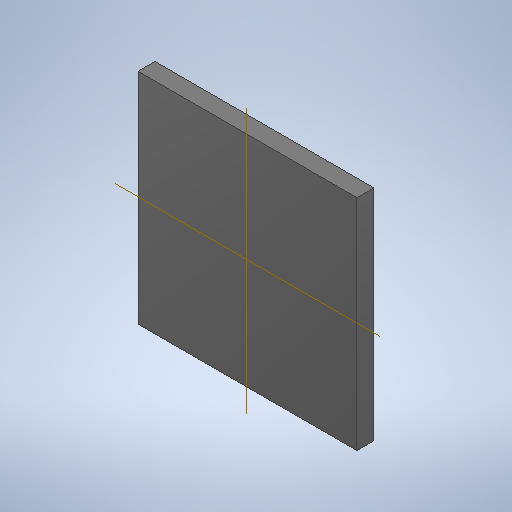
# Autodesk Inventor part: display
Saved by Autodesk Inventor 2025.1 (Build 291241000, 241)
## iProperties
Created: 2024-10-28
Part Number: display
Material: 일반
Document SubType Name: Modeling
Designer: gmsee
Density: 1 g/cm^3
Appearance: 기본값
Author: gmsee
Autodesk Inventor part; units mm, degrees
ref_plane "YZ Plane" through (0, 0, 0) normal (1, 0, 0) x (0, 1, 0)
ref_plane "XZ Plane" through (0, 0, 0) normal (0, 1, 0) x (-1, 0, 0)
ref_plane "XY Plane" through (0, 0, 0) normal (0, 0, 1) x (1, 0, 0)
sketch "스케치1" plane through (0, 0, 0) normal (0, 0, 1) x (1, 0, 0)
  line L0 (-64, 64) -> (65, 64)
  line L1 (65, 64) -> (65, -65)
  line L2 (65, -65) -> (-64, -65)
  line L3 (-64, -65) -> (-64, 64)
  line L4 (0, -90.8) -> (0, 89.8) projected
  line L5 (-89.8, 0) -> (90.8, 0) projected
  point P0 (0, 0)
  dimension "d0" = 129
  dimension "d1" = 129
  dimension "d2" = 64
  dimension "d3" = 64
  constraints: 8 end point, 2 parallel, 1 horizontal, 1 perpendicular
  measures "d0" distance of L0.end L1.end
  measures "d1" distance of L1.end L2.end
  measures "d2" distance between parallel lines of L4 L3
  measures "d3" distance between parallel lines of L5 L0
extrude "돌출1" add sketch "스케치1" against normal blind 10
